LGR RM Carriage Bracket (Goalie) (Autodesk Fusion 360 design; units mm, degrees)
Autodesk Fusion 360 part; units mm, degrees
sketch "Sketch1" plane through (0, 0, 0) normal (0, 0, 1) x (1, 0, 0)
  line L0 (-41, 41) -> (41, 41)
  line L1 (41, 41) -> (41, -41)
  line L2 (41, -41) -> (-41, -41)
  line L3 (-41, -41) -> (-41, 41)
  dimension "d1" = 82
  dimension "d2" = 82
  dimension "d3" = 41
  dimension "d4" = 41
  constraint horizontal L0
  constraint vertical L1
  constraint horizontal L2
  constraint vertical L3
  measures "d1" distance of L1 L3
  measures "d2" distance of L0 L2
  measures "d3" distance of origin L1
  measures "d4" distance of origin L0
extrude "Extrude1" add sketch "Sketch1" along normal blind 6.5
sketch "Sketch2" plane through (0, 0, 6.5) normal (0, 0, 1) x (-1, 0, 0)
  line L0 (41, 41) -> (-41, 41)
  line L1 (-41, 41) -> (-41, -41)
  line L2 (-41, -41) -> (41, -41)
  line L3 (41, -41) -> (41, 41)
  point P0 (34, -30)
  point P1 (-34, -30)
  point P2 (-34, 30)
  point P3 (34, 30)
  dimension "d7" = 68
  dimension "d8" = 60
  dimension "d9" = 7
  dimension "d10" = 11
  constraint horizontal P0 P1
  constraint vertical P1 P2
  constraint horizontal P2 P3
  constraint vertical P0 P3
  measures "d7" distance of P0 P1
  measures "d8" distance of P1 P2
  measures "d9" distance of L1 P1
  measures "d10" distance of L2 P1
hole "Hole1" at (-34, 30, 6.5) at (34, 30, 6.5) at (34, -30, 6.5) at (-34, -30, 6.5) direction (0, 0, -1) diameter 5.5 depth 10 tip angle 180 counterbore diameter 10 counterbore depth 5
sketch "Sketch3" plane through (0, 0, 6.5) normal (0, 0, 1) x (-1, 0, 0)
  circle A0 centre (-34, 30) radius 5
  circle A1 centre (34, -30) radius 5
  circle A2 centre (-34, -30) radius 5
  circle A3 centre (34, 30) radius 5
  line L0 (41, 41) -> (-41, 41)
  line L1 (-41, 41) -> (-41, -41)
  line L2 (-41, -41) -> (41, -41)
  line L3 (41, -41) -> (41, 41)
  line L4 (41, -19.05) -> (-41, -19.05)
  line L5 (-41, -19.05) -> (-41, 19.05)
  line L6 (-41, 19.05) -> (41, 19.05)
  line L7 (41, 19.05) -> (41, -19.05)
  dimension "d16" = 38.1
  dimension "d17" = 19.05
  constraint horizontal L4
  constraint vertical L5
  constraint horizontal L6
  constraint vertical L7
  constraint coincident L1 L5.end
  constraint coincident L3 L4.start
  measures "d16" distance of L4 L6
  measures "d17" distance of origin L6
extrude "Extrude2" cut sketch "Sketch3" against normal blind 4.5 contours L1 L3 L4 L5 L6 L7
fillet "Fillet1" radius 3 2 edges at (0, 19.05, 2) (0, -19.05, 2)
sketch "Sketch4" plane through (0, 0, 6.5) normal (0, 0, 1) x (-1, 0, 0)
  line L0 (41, -19.05) -> (-41, -19.05)
  line L1 (-41, -19.05) -> (-41, -41)
  line L2 (-41, -41) -> (41, -41)
  line L3 (41, -41) -> (41, -19.05)
  circle A0 centre (34, -30) radius 5
  circle A1 centre (-34, -30) radius 5
  line L4 (41, 41) -> (-41, 41)
  line L5 (41, 19.05) -> (41, 41)
  point P0 (-10, -34.75)
  point P1 (10, -34.75)
  point P2 (-10, 34.75)
  point P3 (10, 34.75)
  point P4 (-5.7919, 53.9874)
  dimension "d23" = 6.25
  dimension "d24" = 6.25
  dimension "d25" = 20
  dimension "d26" = 31
  constraint vertical P0 P2
  constraint horizontal P2 P3
  constraint vertical P1 P3
  constraint horizontal P0 P1
  measures "d23" distance of P2 L4
  measures "d24" distance of L2 P0
  measures "d25" distance of P0 P1
  measures "d26" distance of P3 L5
hole "Hole2" at (10, 34.75, 6.5) at (-10, 34.75, 6.5) at (10, -34.75, 6.5) at (-10, -34.75, 6.5) direction (0, 0, -1) diameter 5 end through all
sketch "Sketch7" plane through (0, 0, 6.5) normal (0, 0, 1) x (-1, 0, 0)
  circle A0 centre (-10, 34.75) radius 2.5
  circle A1 centre (10, 34.75) radius 2.5
  line L0 (-41, 19.05) -> (41, 19.05)
  line L1 (41, 19.05) -> (41, 41)
  line L2 (41, 41) -> (-41, 41)
  line L3 (-41, 41) -> (-41, 19.05)
  circle A2 centre (34, 30) radius 5
  circle A3 centre (-34, 30) radius 5
  line L4 (25.5, 22.05) -> (-25.5, 22.05)
  line L5 (-27.5, 24.05) -> (-27.5, 27.05)
  line L6 (-25.5, 29.05) -> (25.5, 29.05)
  line L7 (27.5, 27.05) -> (27.5, 24.05)
  line L8 (25.5, -29.05) -> (-25.5, -29.05)
  line L9 (-27.5, -27.05) -> (-27.5, -24.05)
  line L10 (-25.5, -22.05) -> (25.5, -22.05)
  line L11 (27.5, -24.05) -> (27.5, -27.05)
  line L12 (41, -19.05) -> (-41, -19.05)
  line L13 (-41, -19.05) -> (-41, -41)
  arc A4 (25.5, -29.05) -> (27.5, -27.05) centre (25.5, -27.05) ccw
  arc A5 (27.5, -24.05) -> (25.5, -22.05) centre (25.5, -24.05) ccw
  arc A6 (-25.5, -22.05) -> (-27.5, -24.05) centre (-25.5, -24.05) ccw
  arc A7 (-27.5, -27.05) -> (-25.5, -29.05) centre (-25.5, -27.05) ccw
  arc A8 (25.5, 22.05) -> (27.5, 24.05) centre (25.5, 24.05) ccw
  arc A9 (27.5, 27.05) -> (25.5, 29.05) centre (25.5, 27.05) ccw
  arc A10 (-25.5, 29.05) -> (-27.5, 27.05) centre (-25.5, 27.05) ccw
  arc A11 (-27.5, 24.05) -> (-25.5, 22.05) centre (-25.5, 24.05) ccw
  dimension "d31" = 55
  dimension "d32" = 7
  dimension "d33" = 3
  dimension "d34" = 13.5
  dimension "d35" = 7
  dimension "d36" = 3
  dimension "d37" = 13.5
  dimension "d38" = 55
  dimension "d39" = 2
  constraint horizontal L4
  constraint vertical L5
  constraint horizontal L6
  constraint vertical L7
  constraint horizontal L8
  constraint vertical L9
  constraint horizontal L10
  constraint vertical L11
  constraint tangent L8 A4
  constraint tangent L11 A4
  constraint tangent L11 A5
  constraint tangent L10 A5
  constraint equal A4 A5
  constraint tangent L10 A6
  constraint tangent L9 A6
  constraint equal A4 A6
  constraint tangent L9 A7
  constraint tangent L8 A7
  constraint equal A4 A7
  constraint tangent L4 A8
  constraint tangent L7 A8
  constraint equal A4 A8
  constraint tangent L7 A9
  constraint tangent L6 A9
  constraint equal A4 A9
  constraint tangent L6 A10
  constraint tangent L5 A10
  constraint equal A4 A10
  constraint tangent L5 A11
  constraint tangent L4 A11
  constraint equal A4 A11
  measures "d31" distance of L5 L7
  measures "d32" distance of L4 L6
  measures "d33" distance of L0 L4
  measures "d34" distance of L1 L7
  measures "d35" distance of L8 L10
  measures "d36" distance of L10 L12
  measures "d37" distance of L9 L13
  measures "d38" distance of L9 L11
  measures "d39" radius of A4
extrude "Extrude3" cut sketch "Sketch7" against normal blind 6.5 contours L4 L5 L6 L7 A8 A9 A10 A11 | L8 L9 L10 L11 A4 A5 A6 A7
ref_plane "WorkPlane1" through (0, 0, 6.5) normal (0, 0, -1) x (-1, 0, 0)
sketch "Sketch9" plane through (0, 0, 6.5) normal (0, 0, -1) x (-1, 0, 0)
  line L0 (41, 41) -> (21, 41)
  line L1 (21, 41) -> (21, 37)
  line L2 (21, 37) -> (41, 37)
  line L3 (41, 37) -> (41, 41)
  line L4 (-21, 41) -> (-41, 41)
  line L5 (-41, 41) -> (-41, 37)
  line L6 (-41, 37) -> (-21, 37)
  line L7 (-21, 37) -> (-21, 41)
  line L8 (41, -37) -> (21, -37)
  line L9 (21, -37) -> (21, -41)
  line L10 (21, -41) -> (41, -41)
  line L11 (41, -41) -> (41, -37)
  line L12 (-41, -41) -> (-21, -41)
  line L13 (-21, -41) -> (-21, -37)
  line L14 (-21, -37) -> (-41, -37)
  line L15 (-41, -37) -> (-41, -41)
  point P0 (41, 41)
  dimension "d59" = 82
  dimension "d60" = 82
  dimension "d61" = 4
  dimension "d62" = 20
  dimension "d63" = 20
  dimension "d64" = 4
  dimension "d65" = 20
  dimension "d66" = 20
  dimension "d67" = 4
  dimension "d68" = 4
  constraint horizontal L0
  constraint vertical L1
  constraint horizontal L2
  constraint vertical L3
  constraint horizontal L4
  constraint vertical L5
  constraint horizontal L6
  constraint vertical L7
  constraint horizontal L8
  constraint vertical L9
  constraint horizontal L10
  constraint vertical L11
  constraint horizontal L12
  constraint vertical L13
  constraint horizontal L14
  constraint vertical L15
  constraint vertical P0 L10.end
  constraint horizontal P0 L4.end
  constraint vertical L4.end L12.start
  constraint horizontal L10.end L12.start
  constraint vertical P0 L0.start
  constraint horizontal L0.end P0
  measures "d59" distance of L3 L5
  measures "d60" distance of L0 L10
  measures "d61" distance of L0 L2
  measures "d62" distance of L1 L3
  measures "d63" distance of L5 L7
  measures "d64" distance of L4 L6
  measures "d65" distance of L13 L15
  measures "d66" distance of L9 L11
  measures "d67" distance of L8 L10
  measures "d68" distance of L12 L14
extrude "Extrude5" cut sketch "Sketch9" along normal blind 6.5
fillet "Fillet2" radius 5 4 edges at (-41, 37, 3.25) (41, 37, 3.25) (41, -37, 3.25) (-41, -37, 3.25)
fillet "Fillet3" radius 2 8 edges at (-21, -41, 3.25) (-21, -37, 3.25) (21, -37, 3.25) (21, -41, 3.25) (21, 37, 3.25) (21, 41, 3.25) (-21, 41, 3.25) (-21, 37, 3.25)
sketch "Sketch10" plane through (0, 0, 2) normal (0, 0, 1) x (-1, 0, 0)
  line L0 (41, 16.05) -> (-41, 16.05)
  line L1 (-41, 16.05) -> (-41, -16.05)
  line L2 (-41, -16.05) -> (41, -16.05)
  line L3 (41, -16.05) -> (41, 16.05)
  line L4 (29.8377, -14) -> (-29.8377, -14)
  line L5 (29.8377, 14) -> (-29.8377, 14)
  line L6 (37.5, -10.6064) -> (37.5, 10.6064)
  line L7 (-37.5, -10.6064) -> (-37.5, 10.6064)
  line L8 (41, -19.05) -> (-41, -19.05)
  line L9 (30.154, 12.0513) -> (0.3162, 2.1054)
  line L10 (-0.3162, 2.1054) -> (-30.154, 12.0513)
  line L11 (-36.1798, 11.5537) -> (-4.8025, 0.9473)
  line L12 (-4.8025, -0.9473) -> (-36.1798, -11.5537)
  line L13 (-30.154, -12.0513) -> (-0.3162, -2.1054)
  line L14 (0.3162, -2.1054) -> (30.154, -12.0513)
  line L15 (36.1798, -11.5537) -> (4.8025, -0.9473)
  line L16 (4.8025, 0.9473) -> (36.1798, 11.5537)
  arc A0 (29.8377, -14) -> (30.154, -12.0513) centre (29.8377, -13) ccw
  arc A1 (0.3162, -2.1054) -> (-0.3162, -2.1054) centre (0, -3.0541) ccw
  arc A2 (-30.154, -12.0513) -> (-29.8377, -14) centre (-29.8377, -13) ccw
  arc A3 (-37.5, -10.6064) -> (-36.1798, -11.5537) centre (-36.5, -10.6064) ccw
  arc A4 (-36.1798, 11.5537) -> (-37.5, 10.6064) centre (-36.5, 10.6064) ccw
  arc A5 (-4.8025, -0.9473) -> (-4.8025, 0.9473) centre (-5.1228, 0) ccw
  arc A6 (-0.3162, 2.1054) -> (0.3162, 2.1054) centre (0, 3.0541) ccw
  arc A7 (-29.8377, 14) -> (-30.154, 12.0513) centre (-29.8377, 13) ccw
  arc A8 (30.154, 12.0513) -> (29.8377, 14) centre (29.8377, 13) ccw
  arc A9 (37.5, 10.6064) -> (36.1798, 11.5537) centre (36.5, 10.6064) ccw
  arc A10 (36.1798, -11.5537) -> (37.5, -10.6064) centre (36.5, -10.6064) ccw
  arc A11 (4.8025, 0.9473) -> (4.8025, -0.9473) centre (5.1228, 0) ccw
  point P0 (36, -14)
  point P1 (-36, -14)
  point P2 (-37.5, -12)
  point P3 (-37.5, 12)
  point P4 (0, -2)
  point P5 (-2, 0)
  point P6 (0, 2)
  point P7 (2, 0)
  dimension "d75" = 72
  dimension "d76" = 24
  dimension "d77" = 5
  dimension "d78" = 7.05
  dimension "d79" = 2.05
  dimension "d80" = 2.05
  dimension "d81" = 3.5
  dimension "d82" = 3.5
  dimension "d83" = 1
  constraint parallel L2 L4
  constraint perpendicular L3 L5
  constraint perpendicular L5 L6
  constraint perpendicular L4 L7
  constraint coincident P0 L4
  constraint coincident P0 L14
  constraint tangent L4 A0
  constraint tangent L14 A0
  constraint tangent L14 A1
  constraint tangent L13 A1
  constraint equal A0 A1
  constraint coincident P1 L13
  constraint coincident P1 L4
  constraint tangent L13 A2
  constraint tangent L4 A2
  constraint equal A0 A2
  constraint coincident P2 L12
  constraint coincident P2 L7
  constraint tangent L12 A3
  constraint tangent L7 A3
  constraint equal A0 A3
  constraint coincident P3 L7
  constraint coincident P3 L11
  constraint tangent L7 A4
  constraint tangent L11 A4
  constraint equal A0 A4
  constraint tangent L11 A5
  constraint tangent L12 A5
  constraint equal A0 A5
  constraint tangent L10 A6
  constraint tangent L9 A6
  constraint equal A0 A6
  constraint tangent L10 A7
  constraint tangent L5 A7
  constraint equal A0 A7
  constraint tangent L5 A8
  constraint tangent L9 A8
  constraint equal A0 A8
  constraint tangent L16 A9
  constraint tangent L6 A9
  constraint equal A0 A9
  constraint tangent L6 A10
  constraint tangent L15 A10
  constraint equal A0 A10
  constraint tangent L15 A11
  constraint tangent L16 A11
  constraint equal A0 A11
  measures "d75" distance of P0 P1
  measures "d76" distance of P2 P3
  measures "d77" distance of L1 P1
  measures "d78" distance of P2 L8
  measures "d79" distance of L2 L4
  measures "d80" distance of L0 L5
  measures "d81" distance of L1 L7
  measures "d82" distance of L3 L6
  measures "d83" radius of A0
extrude "Extrude6" cut sketch "Sketch10" against normal blind 2 contours L4 L13 L14 A0 A1 A2 | L5 L9 L10 A6 A7 A8 | L6 L15 L16 A9 A10 A11 | L7 L11 L12 A3 A4 A5
extrude "Extrude7" add 1 faces at (8.5, 16.6833, 0) along direction (0, 0, -1) blind 0.25
extrude "Extrude8" add 2 faces at (41, 10.6667, -0.0833) (41, 27.6732, 3.691) along direction (1, 0, 0) blind 20
sketch "Sketch12" plane through (0, 0, 6.5) normal (0, 0, 1) x (-1, 0, 0)
  arc A0 (-19, 41) -> (-21, 39) centre (-19, 39) ccw
  arc A1 (-23, 37) -> (-21, 39) centre (-23, 39) ccw
  line L0 (-23, 37) -> (-36, 37)
  arc A2 (-36, 37) -> (-41, 32) centre (-36, 32) ccw
  line L1 (-41, 32) -> (-61, 32)
  line L2 (-61, 32) -> (-61, 19.05)
  line L3 (-61, 19.05) -> (41, 19.05)
  line L4 (41, 19.05) -> (41, 32)
  arc A3 (41, 32) -> (36, 37) centre (36, 32) ccw
  line L5 (36, 37) -> (23, 37)
  arc A4 (21, 39) -> (23, 37) centre (23, 39) ccw
  arc A5 (21, 39) -> (19, 41) centre (19, 39) ccw
  line L6 (19, 41) -> (-19, 41)
  circle A6 centre (-34, 30) radius 5
  circle A7 centre (34, 30) radius 5
  circle A8 centre (10, 34.75) radius 2.5
  circle A9 centre (-10, 34.75) radius 2.5
  line L7 (-27.5, 24.05) -> (-27.5, 27.05)
  arc A10 (-25.5, 29.05) -> (-27.5, 27.05) centre (-25.5, 27.05) ccw
  line L8 (-25.5, 29.05) -> (25.5, 29.05)
  arc A11 (27.5, 27.05) -> (25.5, 29.05) centre (25.5, 27.05) ccw
  line L9 (27.5, 27.05) -> (27.5, 24.05)
  arc A12 (25.5, 22.05) -> (27.5, 24.05) centre (25.5, 24.05) ccw
  line L10 (25.5, 22.05) -> (-25.5, 22.05)
  arc A13 (-27.5, 24.05) -> (-25.5, 22.05) centre (-25.5, 24.05) ccw
  line L11 (-61, 32) -> (-41, 32)
  line L12 (-41, 32) -> (-41, 21.05)
  line L13 (-41, 21.05) -> (-61, 21.05)
  line L14 (-61, 21.05) -> (-61, 32)
  line L15 (-61, -32) -> (-41, -32)
  line L16 (-41, -32) -> (-41, -21.05)
  line L17 (-41, -21.05) -> (-61, -21.05)
  line L18 (-61, -21.05) -> (-61, -32)
  line L19 (41, -19.05) -> (-61, -19.05)
  dimension "d90" = 2
  dimension "d91" = 20
  dimension "d92" = 2
  dimension "d93" = 20
  dimension "d94" = 64
  constraint horizontal L11
  constraint vertical L12
  constraint horizontal L13
  constraint vertical L14
  constraint coincident L1.end L2.start
  constraint horizontal L15
  constraint vertical L16
  constraint horizontal L17
  constraint vertical L18
  constraint vertical L1.end L15.start
  measures "d90" distance of L3 L13
  measures "d91" distance of L12 L14
  measures "d92" distance of L17 L19
  measures "d93" distance of L16 L18
  measures "d94" distance of L11 L15
extrude "Extrude9" cut sketch "Sketch12" against normal blind 7 contours L1 L2 L11 L12 L13 L14 | L15 L16 L17 L18
fillet "Fillet4" radius 5 2 edges at (41, 21.05, 3.125) (41, -21.05, 3.125)
fillet "Fillet5" radius 1.5 2 edges at (61, 21.05, 3.125) (61, -21.05, 3.125)
sketch "Sketch14" plane through (0, 0, 2) normal (0, 0, 1) x (-1, 0, 0)
  line L0 (37.5, 10.6064) -> (37.5, -10.6064)
  arc A0 (36.1798, -11.5537) -> (37.5, -10.6064) centre (36.5, -10.6064) ccw
  line L1 (36.1798, -11.5537) -> (4.8025, -0.9473)
  arc A1 (4.8025, 0.9473) -> (4.8025, -0.9473) centre (5.1228, 0) ccw
  line L2 (4.8025, 0.9473) -> (36.1798, 11.5537)
  arc A2 (37.5, 10.6064) -> (36.1798, 11.5537) centre (36.5, 10.6064) ccw
  line L3 (30.154, 12.0513) -> (0.3162, 2.1054)
  arc A3 (-0.3162, 2.1054) -> (0.3162, 2.1054) centre (0, 3.0541) ccw
  line L4 (-0.3162, 2.1054) -> (-30.154, 12.0513)
  arc A4 (-29.8377, 14) -> (-30.154, 12.0513) centre (-29.8377, 13) ccw
  line L5 (-29.8377, 14) -> (29.8377, 14)
  arc A5 (30.154, 12.0513) -> (29.8377, 14) centre (29.8377, 13) ccw
  line L6 (-30.154, -12.0513) -> (-0.3162, -2.1054)
  arc A6 (0.3162, -2.1054) -> (-0.3162, -2.1054) centre (0, -3.0541) ccw
  line L7 (0.3162, -2.1054) -> (30.154, -12.0513)
  arc A7 (29.8377, -14) -> (30.154, -12.0513) centre (29.8377, -13) ccw
  line L8 (29.8377, -14) -> (-29.8377, -14)
  arc A8 (-30.154, -12.0513) -> (-29.8377, -14) centre (-29.8377, -13) ccw
  line L9 (-4.8025, -0.9473) -> (-36.1798, -11.5537)
  arc A9 (-37.5, -10.6064) -> (-36.1798, -11.5537) centre (-36.5, -10.6064) ccw
  line L10 (-37.5, -10.6064) -> (-37.5, 10.6064)
  arc A10 (-36.1798, 11.5537) -> (-37.5, 10.6064) centre (-36.5, 10.6064) ccw
  line L11 (-36.1798, 11.5537) -> (-4.8025, 0.9473)
  arc A11 (-4.8025, -0.9473) -> (-4.8025, 0.9473) centre (-5.1228, 0) ccw
  line L12 (41, 16.05) -> (-61, 16.05)
  line L13 (-61, 16.05) -> (-61, -16.05)
  line L14 (-61, -16.05) -> (41, -16.05)
  line L15 (41, -16.05) -> (41, 16.05)
  line L16 (-57.5, 10.5218) -> (-57.5, -10.5218)
  line L17 (-41, 10.5218) -> (-41, -10.5218)
  line L18 (-41.94, -10.7593) -> (-47.2368, -0.9503)
  line L19 (-47.2368, 0.9503) -> (-41.94, 10.7593)
  line L20 (-56.56, 10.7593) -> (-51.2632, 0.9503)
  line L21 (-51.2632, -0.9503) -> (-56.56, -10.7593)
  line L22 (-55.0268, 14) -> (-43.4732, 14)
  line L23 (-42.6049, 12.5039) -> (-48.3818, 2.3944)
  line L24 (-50.1182, 2.3944) -> (-55.8951, 12.5039)
  line L25 (-55.8951, -12.5039) -> (-50.1182, -2.3944)
  line L26 (-48.3818, -2.3944) -> (-42.6049, -12.5039)
  line L27 (-43.4732, -14) -> (-55.0268, -14)
  arc A12 (-55.0268, 14) -> (-55.8951, 12.5039) centre (-55.0268, 13) ccw
  arc A13 (-42.6049, 12.5039) -> (-43.4732, 14) centre (-43.4732, 13) ccw
  arc A14 (-55.8951, -12.5039) -> (-55.0268, -14) centre (-55.0268, -13) ccw
  arc A15 (-43.4732, -14) -> (-42.6049, -12.5039) centre (-43.4732, -13) ccw
  arc A16 (-48.3818, -2.3944) -> (-50.1182, -2.3944) centre (-49.25, -2.8906) ccw
  arc A17 (-50.1182, 2.3944) -> (-48.3818, 2.3944) centre (-49.25, 2.8906) ccw
  arc A18 (-41, 10.5218) -> (-41.94, 10.7593) centre (-41.5, 10.5218) ccw
  arc A19 (-41.94, -10.7593) -> (-41, -10.5218) centre (-41.5, -10.5218) ccw
  arc A20 (-57.5, -10.5218) -> (-56.56, -10.7593) centre (-57, -10.5218) ccw
  arc A21 (-51.2632, -0.9503) -> (-51.2632, 0.9503) centre (-53.023, 0) ccw
  arc A22 (-47.2368, 0.9503) -> (-47.2368, -0.9503) centre (-45.477, 0) ccw
  arc A23 (-56.56, 10.7593) -> (-57.5, 10.5218) centre (-57, 10.5218) ccw
  point P0 (-57.5, 12.5)
  point P1 (-57.5, -12.5)
  point P2 (-47.75, 0)
  point P3 (-50.75, 0)
  point P4 (-49.25, 0.875)
  point P5 (-56.75, -14)
  point P6 (-49.25, -0.875)
  point P7 (-41.75, -14)
  dimension "d106" = 3.5
  dimension "d107" = 3.5
  dimension "d108" = 2.05
  dimension "d109" = 2.05
  dimension "d110" = 25
  dimension "d111" = 12.5
  dimension "d112" = 15
  dimension "d113" = 0.75
  dimension "d114" = 3
  dimension "d115" = 1.75
  dimension "d116" = 1.5
  dimension "d117" = 0.875
  dimension "d118" = 8.25
  dimension "d119" = 1
  dimension "d120" = 0.5
  dimension "d121" = 2
  dimension "d122" = 0.5
  constraint vertical L16
  constraint perpendicular L12 L17
  constraint perpendicular L16 L22
  constraint horizontal P2 P3
  constraint vertical P4 P6
  constraint horizontal origin P2
  constraint tangent L24 A12
  constraint tangent L22 A12
  constraint tangent L22 A13
  constraint tangent L23 A13
  constraint equal A12 A13
  constraint coincident P5 L25
  constraint coincident P5 L27
  constraint tangent L25 A14
  constraint tangent L27 A14
  constraint equal A12 A14
  constraint coincident P7 L27
  constraint coincident P7 L26
  constraint tangent L27 A15
  constraint tangent L26 A15
  constraint equal A12 A15
  constraint coincident P6 L26
  constraint coincident P6 L25
  constraint tangent L26 A16
  constraint tangent L25 A16
  constraint equal A12 A16
  constraint coincident P4 L24
  constraint coincident P4 L23
  constraint tangent L24 A17
  constraint tangent L23 A17
  constraint equal A12 A17
  constraint tangent L19 A18
  constraint tangent L17 A18
  constraint tangent L17 A19
  constraint tangent L18 A19
  constraint equal A18 A19
  constraint coincident P1 L21
  constraint coincident P1 L16
  constraint tangent L21 A20
  constraint tangent L16 A20
  constraint equal A18 A20
  constraint coincident P3 L20
  constraint coincident P3 L21
  constraint tangent L20 A21
  constraint tangent L21 A21
  constraint coincident P2 L18
  constraint coincident P2 L19
  constraint tangent L18 A22
  constraint tangent L19 A22
  constraint equal A21 A22
  constraint coincident P0 L16
  constraint coincident P0 L20
  constraint tangent L16 A23
  constraint tangent L20 A23
  measures "d106" distance of L13 L16
  measures "d107" distance of L10 L17
  measures "d108" distance of L12 L22
  measures "d109" distance of L14 L27
  measures "d110" distance of P0 P1
  measures "d111" vertical distance of origin P0
  measures "d112" distance of P5 P7
  measures "d113" horizontal distance of P1 P5
  measures "d114" distance of P2 P3
  measures "d115" distance of P4 P6
  measures "d116" horizontal distance of P3 P4
  measures "d117" vertical distance of P2 P6
  measures "d118" distance of L17 P4
  measures "d119" radius of A12
  measures "d120" radius of A18
  measures "d121" radius of A21
  measures "d122" radius of A23
extrude "Extrude11" cut sketch "Sketch14" against normal blind 3 contours L16 L20 L21 A20 A21 A23 | L17 L18 L19 A18 A19 A22 | L22 L23 L24 A12 A13 A17 | L25 L26 L27 A14 A15 A16
equation "d3 = ( 82 / 2 ) * 1 mm"
equation "d4 = ( 82 / 2 ) * 1 mm"
equation "d9 = ( ( 82 - 68 ) / 2 ) * 1 mm"
equation "d10 = ( ( 82 - 60 ) / 2 ) * 1 mm"
equation "d17 = ( 38.1 / 2 ) * 1 mm"
equation "d26 = ( ( 82 - 20 ) / 2 ) * 1 mm"
equation "d34 = ( ( 82 - 55 ) / 2 ) * 1 mm"
equation "d37 = ( ( 82 - 55 ) / 2 ) * 1 mm"
equation "d77 = ( ( 82 - 72 ) / 2 ) * 1 mm"
equation "d78 = ( ( 38.1 - 24 ) / 2 ) * 1 mm"
equation "d113 = ( ( 16.5 - 15 ) / 2 ) * 1 mm"
equation "d117 = ( 1.75 / 2 ) * 1 mm"
equation "d118 = ( 16.5 / 2 ) * 1 mm"
